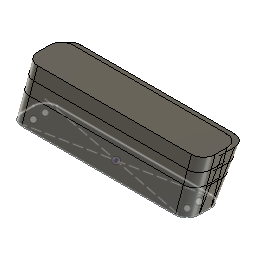
ID3_Wireless_Charger_Offsetter (Autodesk Fusion 360 design; units mm, degrees)
part number: 2026-05-14-21-16-16-343
Autodesk Fusion 360 part; units mm, degrees
sketch "Base" plane through (0, 0, 0) normal (0, 0, 1) x (1, 0, 0)
  line L0 (32.5, 7.5) -> (-32.5, 7.5)
  line L1 (-37.5, 2.5) -> (-37.5, -2.5)
  line L2 (-32.5, -7.5) -> (32.5, -7.5)
  line L3 (37.5, -2.5) -> (37.5, 2.5)
  line L4 (37.5, 7.5) -> (-37.5, -7.5) construction
  line L5 (-37.5, 7.5) -> (37.5, -7.5) construction
  arc A0 (-32.5, 7.5) -> (-37.5, 2.5) centre (-32.5, 2.5) ccw
  arc A1 (-37.5, -2.5) -> (-32.5, -7.5) centre (-32.5, -2.5) ccw
  arc A2 (32.5, -7.5) -> (37.5, -2.5) centre (32.5, -2.5) ccw
  arc A3 (37.5, 2.5) -> (32.5, 7.5) centre (32.5, 2.5) ccw
  dimension "d1" = 75
  dimension "d2" = 15
  dimension "d3" = 5
  dimension "d4" = 5
  constraint horizontal L0
  constraint perpendicular L0 L1
  constraint parallel L0 L2
  constraint parallel L1 L3
  constraint coincident L4 origin
  constraint coincident L5 origin
  constraint coincident L5.start L0
  constraint coincident L5.start L1
  constraint tangent L0 A0
  constraint tangent L1 A0
  constraint coincident L4.end L2
  constraint coincident L4.end L1
  constraint tangent L2 A1
  constraint tangent L1 A1
  constraint coincident L5.end L2
  constraint coincident L5.end L3
  constraint tangent L2 A2
  constraint tangent L3 A2
  constraint equal A1 A2
  constraint coincident L4.start L3
  constraint coincident L4.start L0
  constraint tangent L3 A3
  constraint tangent L0 A3
  constraint equal A1 A3
  measures "d1" distance of L4.end L5.end
  measures "d2" distance of L5.start L4.end
  measures "d3" radius of A0
  measures "d4" radius of A1
ref_plane "WorkPlane1" through (0, -7.5, 0) normal (0, -0.939693, 0.34202) x (1, 0, 0)
sketch "20mm20deg" plane through (0, -6.6227, 2.4105) normal (0, -0.939693, 0.34202) x (1, 0, 0)
  line L0 (0, 0) -> (0, 20)
  dimension "d6" = 20
  constraint coincident L0.start origin
  constraint vertical L0
  measures "d6" distance of L0.start L0.end
sweep "Sweep1" add profiles "Base" path "20mm20deg" along L0 section 1 makes body 1
sketch "15mm20deg" plane through (0, -6.6227, 2.4105) normal (0, -0.939693, 0.34202) x (1, 0, 0)
  line L0 (0, 0) -> (0, 15)
  dimension "d13" = 15
  constraint coincident L0.start origin
  constraint vertical L0
  measures "d13" distance of L0.start L0.end
sweep "Sweep2" add profiles "Base" path "15mm20deg" along L0 section 1 separate body makes body 2
sketch "10mm20deg" plane through (0, -6.6227, 2.4105) normal (0, -0.939693, 0.34202) x (1, 0, 0)
  line L0 (0, 0) -> (0, 10)
  dimension "d20" = 10
  constraint coincident L0.start origin
  constraint vertical L0
  measures "d20" distance of L0.start L0.end
sweep "Sweep3" add profiles "Base" path "10mm20deg" along L0 section 1 separate body makes body 3
ref_plane "WorkPlane2" through (0, -7.5, 0) normal (0, -0.866025, 0.5) x (1, 0, 0)
sketch "20mm30deg" plane through (0, -5.625, 3.2476) normal (0, -0.866025, 0.5) x (1, 0, 0)
  line L0 (0, 0) -> (0, 20)
  dimension "d28" = 20
  constraint coincident L0.start origin
  constraint vertical L0
  measures "d28" distance of L0.start L0.end
sketch "15mm30deg" plane through (0, -5.625, 3.2476) normal (0, -0.866025, 0.5) x (1, 0, 0)
  line L0 (0, 0) -> (0, 15)
  dimension "d29" = 15
  constraint coincident L0.start origin
  constraint vertical L0
  measures "d29" distance of L0.start L0.end
sketch "10mm30deg" plane through (0, -5.625, 3.2476) normal (0, -0.866025, 0.5) x (1, 0, 0)
  line L0 (0, 0) -> (0, 10)
  dimension "d30" = 10
  constraint coincident L0.start origin
  constraint vertical L0
  measures "d30" distance of L0.start L0.end
sweep "Sweep4" add profiles "Base" path "10mm30deg" along L0 section 1 separate body makes body 4
sweep "Sweep5" add profiles "Base" path "15mm30deg" along L0 section 1 separate body makes body 5
sweep "Sweep6" add profiles "Base" path "20mm30deg" along L0 section 1 separate body makes body 6
named bodies: "20mm20deg", "15mm20deg", "10mm20deg", "10mm30deg", "15mm30deg", "20mm30deg"
